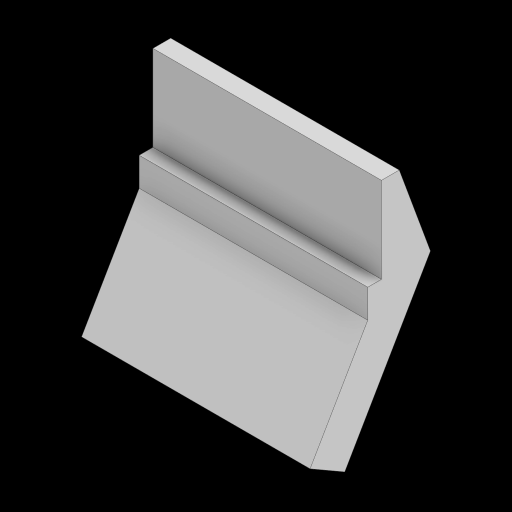
# Autodesk Inventor part: ANS9-2-BK
Saved by Autodesk Inventor 2024 (Build 280153000, 153)
## iProperties
Created: 2023-10-29
Part Number: ANS9-2-BK
Material: Generic
Document SubType Name: Modeling
Designer: bennk
Density: 1 g/cm^3
Appearance: Default
Author: bennk
Autodesk Inventor part; units mm, degrees
ref_plane "YZ Plane" through (0, 0, 0) normal (1, 0, 0) x (0, 1, 0)
ref_plane "XZ Plane" through (0, 0, 0) normal (0, 1, 0) x (-1, 0, 0)
ref_plane "XY Plane" through (0, 0, 0) normal (0, 0, 1) x (1, 0, 0)
sketch "Sketch1" plane through (0, 0, 0) normal (1, 0, 0) x (0, 1, 0)
  line L0 (0, 0) -> (-32.9956, 19.05)
  line L1 (-32.9956, 19.05) -> (-28.5506, 26.749)
  line L2 (-28.5506, 26.749) -> (-6.35, 13.9315)
  line L3 (-6.35, 13.9315) -> (0, 13.9315)
  line L4 (0, 13.9315) -> (0, 10.8835)
  line L5 (0, 10.8835) -> (19.05, 10.8835)
  line L6 (19.05, 10.8835) -> (19.05, 6.9336)
  line L7 (19.05, 6.9336) -> (0, 0)
  dimension "d0" = 38.1
  dimension "d1" = 8.89
  dimension "d2" = 30
  dimension "d3" = 19.05
  dimension "d5" = 3.048
  dimension "d6" = 20
  dimension "d7" = 6.35
  constraints: 16 end point, 4 perpendicular, 1 horizontal, 1 point on line, 1 vertical
  measures "d0" distance of L0.start L0.end
  measures "d1" distance of L0.end L1.end
  measures "d2" angle of L3 L2
  measures "d3" distance of L4.end L5.end
  measures "d5" distance of L3.end L4.end
  measures "d6" angle of L7 L5
  measures "d7" distance of L2.end L3.end
extrude "Extrusion1" add sketch "Sketch1" along normal blind 50.8
body "Solid1"
